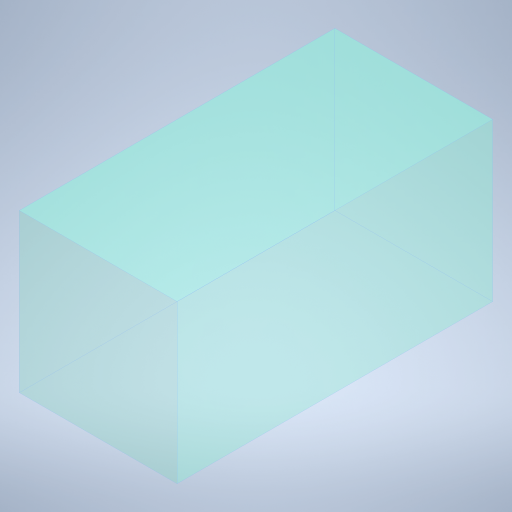
# Autodesk Inventor part: WaterAndBoatLimit
Saved by Autodesk Inventor 2024 (Build 280153000, 153)
## iProperties
Created: 2023-06-12
Part Number: WaterAndBoatLimit
Material: Water
Document SubType Name: Modeling
Designer: 18179
Density: 0.9983 g/cm^3
Appearance: Tropical Blue
Author: 18179
Autodesk Inventor part; units mm, degrees
ref_plane "YZ Plane" through (0, 0, 0) normal (1, 0, 0) x (0, 1, 0)
ref_plane "XZ Plane" through (0, 0, 0) normal (0, 1, 0) x (-1, 0, 0)
ref_plane "XY Plane" through (0, 0, 0) normal (0, 0, 1) x (1, 0, 0)
sketch "Sketch1" plane through (0, 0, 0) normal (0, 0, 1) x (1, 0, 0)
  line L0 (0, 0) -> (-914.4, 0)
  line L1 (-914.4, 0) -> (-914.4, 914.4)
  line L2 (-914.4, 914.4) -> (0, 914.4)
  line L3 (0, 914.4) -> (0, 0)
  dimension "d0" = 914.4
  dimension "d1" = 914.4
  constraints: 8 end point, 2 parallel, 1 horizontal, 1 perpendicular
  measures "d0" distance of L1.end L2.end
  measures "d1" distance of L0.end L1.end
extrude "Extrusion1" add sketch "Sketch1" along normal blind 1828.8
body "Solid1"
